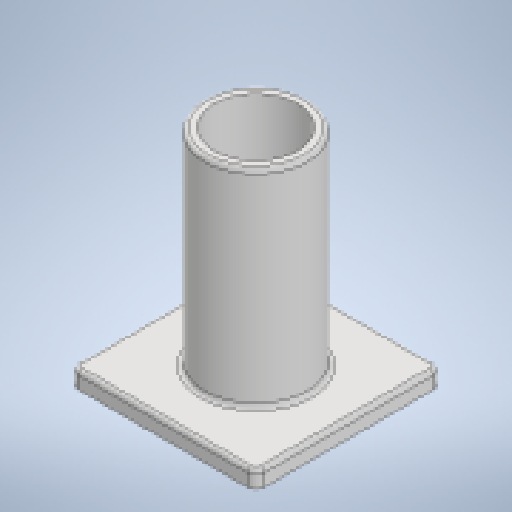
# Autodesk Inventor part: pole-2
Saved by Autodesk Inventor 2025 (Build 290162000, 162)
## iProperties
Created: 2026-01-29
Part Number: pole-2
Material: 一般
Document SubType Name: Modeling
Designer: mahhy
Density: 1 g/cm^3
Appearance: 既定
Author: mahhy
## iProperties of the stored document pole-2_3D プリント.ipt
Created: 2026-01-29
Part Number: pole-2_3D プリント
Material: 一般
Document SubType Name: Modeling
Designer: mahhy
Density: 1 g/cm^3
Appearance: 既定
Author: mahhy
Autodesk Inventor part; units mm, degrees
ref_plane "YZ Plane" through (0, 0, 0) normal (1, 0, 0) x (0, 1, 0)
ref_plane "XZ Plane" through (0, 0, 0) normal (0, 1, 0) x (-1, 0, 0)
ref_plane "XY Plane" through (0, 0, 0) normal (0, 0, 1) x (1, 0, 0)
sketch "底面" plane through (0, 0, 0) normal (0, 1, 0) x (-1, 0, 0)
  line L0 (2, 0) -> (43, 0)
  line L1 (45, -2) -> (45, -43)
  line L2 (43, -45) -> (2, -45)
  line L3 (0, -43) -> (0, -2)
  arc A0 (45, -2) -> (43, 0) centre (43, -2) ccw
  arc A1 (43, -45) -> (45, -43) centre (43, -43) ccw
  arc A2 (0, -43) -> (2, -45) centre (2, -43) ccw
  arc A3 (2, 0) -> (0, -2) centre (2, -2) ccw
  circle A4 centre (22.5, -22.5) radius 10
  point P0 (0, 0)
  point P1 (45, -45)
  point P2 (45, 0)
  point P3 (0, -45)
  point P4 (45, -22.5)
  point P5 (22.5, 0)
  dimension "d0" = 45
  dimension "d1" = 45
  dimension "d2" = 2
  dimension "d8" = 20
  constraints: 8 end point, 8 point on circle, 8 point on line, 8 tangent, 5 centre point, 3 equal radius, 2 midpoint, 2 parallel, 1 horizontal, 1 horizontal alignment, 1 perpendicular, 1 vertical alignment
  measures "d0" distance of point (45, -45) point (0, -45)
  measures "d1" distance of point (45, 0) point (45, -45)
  measures "d2" radius of A0
  measures "d8" diameter of A4
extrude "底" add sketch "底面" along normal blind 4
sketch "スケッチ2" plane through (0, 4, 0) normal (0, 1, 0) x (1, 0, 0)
  circle A0 centre (-22.5, 22.5) radius 12.5
  line L0 (-43, 0) -> (-2, 0) projected
  line L1 (-45, 43) -> (-45, 2) projected
  circle A1 centre (-22.5, 22.5) radius 10 projected
  point P0 (0, 0)
  point P1 (-22.5, 0)
  point P2 (-45, 22.5)
  dimension "d5" = 25
  constraints: 2 midpoint, 1 centre point, 1 horizontal alignment, 1 vertical alignment
  measures "d5" diameter of A0
extrude "棒" add sketch "スケッチ2" along normal blind 50
fillet "フィレット1" radius 1 2 edges at (-35, 4, -22.5) (-35, 54, -22.5)
fillet "フィレット2" radius 1 8 edges at (-0.5858, 4, -0.5858) (0, 4, -22.5) (-0.5858, 4, -44.4142) (-22.5, 4, -45) (-44.4142, 4, -44.4142) (-45, 4, -22.5) (-44.4142, 4, -0.5858) (-22.5, 4, 0)
equation "\"d0\" = d1"
